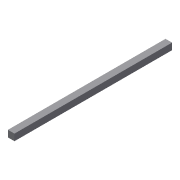
# Autodesk Inventor part: clawBase
Saved by Autodesk Inventor 2015 (Build 190159000, 159)
## iProperties
Created: 2015-01-13
Part Number: clawBase
Material: Generic
Document SubType Name: Modeling
Designer: Collin_2
Density: 1 g/cm^3
Appearance: Default
Author: Collin_2
Autodesk Inventor part; units mm, degrees
ref_plane "YZ Plane" through (0, 0, 0) normal (1, 0, 0) x (0, 1, 0)
ref_plane "XZ Plane" through (0, 0, 0) normal (0, 1, 0) x (-1, 0, 0)
ref_plane "XY Plane" through (0, 0, 0) normal (0, 0, 1) x (1, 0, 0)
sketch "Sketch1" plane through (0, 0, 0) normal (0, 1, 0) x (-1, 0, 0)
  line L0 (49.7782, 121.4529) -> (24.3782, 121.4529)
  line L1 (24.3782, 121.4529) -> (24.3782, -488.1471)
  line L2 (24.3782, -488.1471) -> (49.7782, -488.1471)
  line L3 (49.7782, -488.1471) -> (49.7782, 121.4529)
  point P0 (0, 0)
  dimension "d0" = 25.4
  dimension "d1" = 609.6
  constraints: 8 end point, 2 parallel, 1 horizontal, 1 perpendicular
  measures "d0" distance of L0.start L0.end
  measures "d1" distance of L2.end L0.start
extrude "Extrusion1" add sketch "Sketch1" along normal blind 25.4
body "Solid1"
